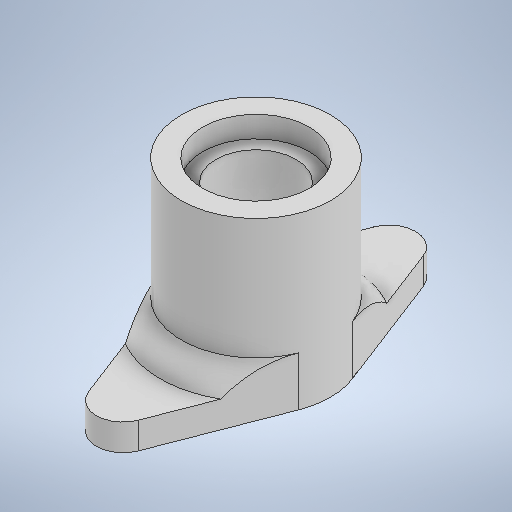
# Autodesk Inventor part: Quiz1
Saved by Autodesk Inventor 2025.2 (Build 292293000, 293)
## iProperties
Created: 2024-11-28
Part Number: Quiz1
Material: Generic
Document SubType Name: Modeling
Designer: hongquan
Density: 1 g/cm^3
Appearance: Default
Author: hongquan
Autodesk Inventor part; units mm, degrees
ref_plane "YZ Plane" through (0, 0, 0) normal (1, 0, 0) x (0, 1, 0)
ref_plane "XZ Plane" through (0, 0, 0) normal (0, 1, 0) x (-1, 0, 0)
ref_plane "XY Plane" through (0, 0, 0) normal (0, 0, 1) x (1, 0, 0)
sketch "Sketch1" plane through (0, 0, 0) normal (1, 0, 0) x (0, 1, 0)
  line L0 (119.9441, 0) -> (-107.8442, 0)
  line L1 (140, -37.5) -> (140, -50)
  line L2 (140, -50) -> (160, -50)
  line L3 (160, -50) -> (160, -70)
  line L4 (31.9465, -37.5) -> (140, -37.5)
  line L5 (0, -150) -> (25, -150)
  line L6 (25, -150) -> (25, -90)
  line L7 (0, 154.1092) -> (0, 150) construction
  line L8 (0, -70) -> (0, -195.8423) construction
  line L9 (0, -70) -> (0, -150)
  line L10 (25, -150) -> (25, -90)
  line L11 (160, -70) -> (46.487, -70)
  line L12 (0.0098, -70) -> (0, -70)
  arc A0 (25, -90) -> (46.487, -70) centre (-38.72, 0) ccw
  arc A1 (0, -70.0054) -> (31.9465, -37.5) centre (-38.72, 0) ccw
  point P0 (0, 0)
  point P1 (150, -50)
  point P2 (18.337, -56.0758)
  dimension "d0" = 20
  dimension "d2" = 100
  dimension "d4" = 75
  dimension "d7" = 38.72
  dimension "d8" = 300
  dimension "d9" = 25
  dimension "d10" = 60
  dimension "d11" = 160
  dimension "d12" = 140
  constraints: 26 end point, 12 perpendicular, 6 point on circle, 5 vertical, 3 horizontal, 2 centre point, 2 point on line, 1 coincident, 1 midpoint, 1 other
  measures "d0" distance of L1.end L2.end
  measures "d2" diameter of point (150, -50) L0
  measures "d4" diameter of L4 L0
  measures "d7" distance of A1.centre point (0, 0)
  measures "d8" distance of L7.end L5.start
  measures "d9" distance of L5.start L5.end
  measures "d10" distance of L6.end L5.end
  measures "d11" distance between parallel lines of L9 L3
  measures "d12" diameter of L11 L0
revolve "Revolution1" add sketch "Sketch1" angle 360 about axis through (0, 119.9441, 0) along (0, -1, 0) contours L1 L2 L3 L11 A0 L6 L5 L9 A1 L4
sketch "Sketch2" plane through (0, 25, 0) normal (0, 1, 0) x (1, 0, 0)
  circle A0 centre (0, -120) radius 12.5
  arc A1 (-23.3236, -133.9943) -> (23.3236, -133.9943) centre (0, -124.9939) ccw
  line L0 (0, 213.9519) -> (0, -189.1435) construction
  circle A2 centre (0, 0) radius 70
  circle A3 centre (0, 0) radius 70 projected
  line L1 (216.3498, 0) -> (-212.0735, 0)
  circle A4 centre (0, 120) radius 12.5
  arc A5 (23.3236, 133.9943) -> (-23.3236, 133.9943) centre (0, 124.9939) ccw
  line L2 (-23.3236, 133.9943) -> (-65.3062, 25.2012)
  line L3 (-100.3964, -65.731) -> (-103.3588, -73.4078)
  line L4 (-23.3236, -133.9943) -> (-65.3062, -25.2012)
  line L5 (-100.3964, 65.731) -> (-103.3588, 73.4078)
  line L6 (23.3236, 133.9943) -> (65.3062, 25.2012)
  line L7 (100.3964, -65.731) -> (103.3588, -73.4078)
  line L8 (23.3236, -133.9943) -> (65.3062, -25.2012)
  line L9 (100.3964, 65.731) -> (103.3588, 73.4078)
  arc A6 (30.216, -116.1335) -> (30.216, 116.1335) centre (0, 0) ccw
  arc A7 (-30.216, 116.1335) -> (-30.216, -116.1335) centre (0, 0) ccw
  circle A8 centre (0, 0) radius 150.0812
  point P0 (0, -149.9939)
  point P1 (0, -120)
  point P2 (-18.02, -147.7381)
  point P3 (18.02, -147.7381)
  point P4 (-18.02, 147.7381)
  point P5 (18.02, 147.7381)
  dimension "d16" = 25
  dimension "d17" = 50
  constraints: 20 end point, 17 point on circle, 8 centre point, 8 symmetric about line, 7 point on line, 5 coincident, 4 tangent, 2 horizontal, 2 vertical, 7 other
  measures "d16" diameter of A0
  measures "d17" diameter of A1
extrude "Extrusion1" cut sketch "Sketch2" along normal blind 25 and the other way blind 25 contours A1 L8 A6 L1 A8 A7 L4 | A7 L1 A2 L4 | L8 A2 L1 A6 | L1 A7 L2 A2 | L1 A8 A6 L6 A5 L2 A7 | A2 L6 A6 L1
body "Solid1"
